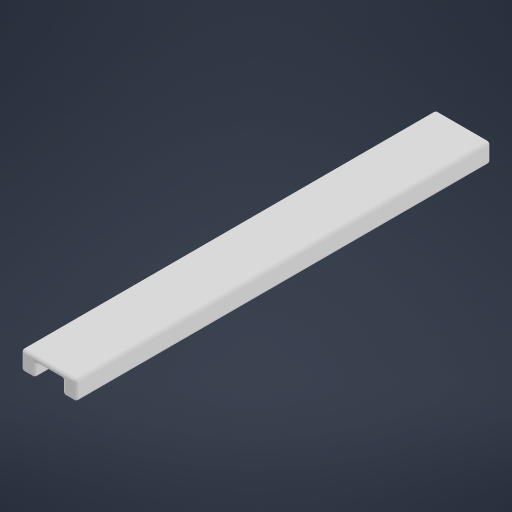
# Autodesk Inventor part: Cable_Cover
Saved by Autodesk Inventor 2024 (Build 280153000, 153)
## iProperties
Created: 2023-07-08
Part Number: Cable_Cover
Material: Generic
Document SubType Name: Modeling
Designer: User
Density: 1 g/cm^3
Appearance: Default
Author: User
Autodesk Inventor part; units mm, degrees
ref_plane "YZ Plane" through (0, 0, 0) normal (1, 0, 0) x (0, 1, 0)
ref_plane "XZ Plane" through (0, 0, 0) normal (0, 1, 0) x (-1, 0, 0)
ref_plane "XY Plane" through (0, 0, 0) normal (0, 0, 1) x (1, 0, 0)
sketch "Sketch3" plane through (0, 0, 0) normal (0, 0, 1) x (1, 0, 0)
  line L0 (0, 0) -> (0, 7)
  line L1 (0, 7) -> (-20, 7)
  line L2 (-20, 7) -> (-20, 0)
  line L3 (-20, 0) -> (-15, 0)
  line L4 (-15, 0) -> (-15, 5)
  line L5 (-15, 5) -> (-5, 5)
  line L6 (-15, 5) -> (-5, 5) construction
  line L7 (-5, 5) -> (-5, 0)
  line L8 (-5, 0) -> (0, 0)
  dimension "d22" = 7
  dimension "d23" = 20
  dimension "d24" = 90
  dimension "d25" = 7
  dimension "d26" = 90
  dimension "d27" = 5
  dimension "d28" = 90
  dimension "d29" = 5
  dimension "d30" = 10
  dimension "d31" = 0
  dimension "d32" = 5
  dimension "d33" = 90
  constraints: 18 end point, 5 perpendicular, 2 horizontal, 1 collinear, 1 vertical
  measures "d22" distance of L0.start L0.end
  measures "d23" distance of L0.end L1.end
  measures "d24" angle of L1 L0
  measures "d25" distance of L1.end L2.end
  measures "d26" angle of L2 L1
  measures "d27" distance of L2.end L3.end
  measures "d28" angle of L3 L2
  measures "d29" distance of L3.end L4.end
  measures "d30" distance of L4.end L5.end
  measures "d31" distance between parallel lines of L5 L6
  measures "d32" distance of L5.end L7.end
  measures "d33" angle of L5 L7
extrude "Extrusion3" add sketch "Sketch3" along normal blind 150
fillet "Fillet4" radius 1 20 edges at (-15, 2.5, 150) (-10, 5, 150) (-5, 2.5, 150) (-5, 2.5, 0) (-5, 0, 75) (-2.5, 0, 150) (0, 3.5, 150) (0, 0, 75) (0, 3.5, 0) (-10, 7, 150) (-20, 3.5, 150) (-17.5, 0, 150) (-15, 0, 75) (-15, 2.5, 0) (-20, 3.5, 0) (-20, 0, 75) (-10, 7, 0) (-10, 5, 0) (-2.5, 0, 0) (-17.5, 0, 0)
fillet "Fillet5" radius 1 2 edges at (-4.7071, 5.2929, 149.7071) (-15.2929, 5.2929, 149.7071)
fillet "Fillet6" radius 1 6 edges at (-0.2929, 6.7071, 149.7071) (-0.2929, 6.7071, 0.2929) (0, 7, 75) (-19.7071, 6.7071, 149.7071) (-19.7071, 6.7071, 0.2929) (-20, 7, 75)
body "Solid2"
